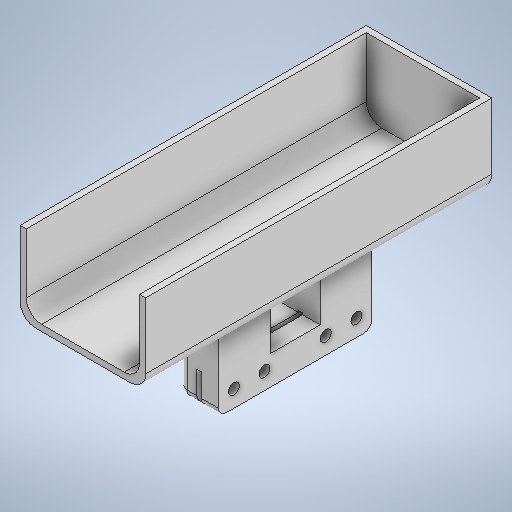
# Autodesk Inventor part: Battery and Rotation Sensor Holder
Saved by Autodesk Inventor 2025.1 (Build 291241020, 241B)
## iProperties
Created: 2024-12-11
Part Number: Battery and Rotation Sensor Holder
Material: Generic
Document SubType Name: Modeling
Designer: AtuStem
Density: 1 g/cm^3
Appearance: Default
Author: AtuStem
Autodesk Inventor part; units mm, degrees
ref_plane "YZ Plane" through (0, 0, 0) normal (1, 0, 0) x (0, 1, 0)
ref_plane "XZ Plane" through (0, 0, 0) normal (0, 1, 0) x (-1, 0, 0)
ref_plane "XY Plane" through (0, 0, 0) normal (0, 0, 1) x (1, 0, 0)
sketch "Sketch1" plane through (0, 0, 0) normal (1, 0, 0) x (0, 1, 0)
  line L0 (0, 0) -> (0, -12.7)
  circle A0 centre (0, -12.7) radius 3.9624
  line L1 (-6.985, -31.75) -> (5.08, -31.75)
  line L2 (5.08, -31.75) -> (5.08, 0)
  line L3 (5.08, 0) -> (-6.985, 0)
  line L4 (-6.985, 0) -> (-6.985, -31.75)
  circle A1 centre (0, -25.4) radius 3.9624
  line L5 (5.08, -10.3505) -> (29.6164, -10.3505)
  line L6 (29.6164, -10.3505) -> (29.6164, -31.75)
  line L7 (29.6164, -31.75) -> (5.08, -31.75)
  line L8 (5.08, -31.75) -> (5.08, -10.3505)
  line L9 (29.6164, -71.755) -> (27.0764, -71.755)
  line L10 (27.0764, -71.755) -> (27.0764, 0)
  line L11 (27.0764, 0) -> (29.6164, 0)
  line L12 (29.6164, 0) -> (29.6164, -71.755)
  line L13 (0, 0) -> (0, 12.7)
  circle A2 centre (0, 12.7) radius 3.9624
  line L14 (-6.985, 31.75) -> (5.08, 31.75)
  line L15 (5.08, 31.75) -> (5.08, 0)
  line L16 (-6.985, 0) -> (-6.985, 31.75)
  circle A3 centre (0, 25.4) radius 3.9624
  line L17 (5.08, 10.3505) -> (29.6164, 10.3505)
  line L18 (29.6164, 10.3505) -> (29.6164, 31.75)
  line L19 (29.6164, 31.75) -> (5.08, 31.75)
  line L20 (5.08, 31.75) -> (5.08, 10.3505)
  line L21 (29.6164, 71.755) -> (27.0764, 71.755)
  line L22 (27.0764, 71.755) -> (27.0764, 0)
  line L23 (29.6164, 0) -> (29.6164, 71.755)
  circle A4 centre (0, -25.4) radius 2.286
  circle A5 centre (0, -12.7) radius 2.286
  circle A6 centre (0, 12.7) radius 2.286
  circle A7 centre (0, 25.4) radius 2.286
  point P0 (27.0764, -31.75)
  point P1 (27.0764, -10.3505)
  point P2 (27.0764, 10.3505)
  point P3 (27.0764, 31.75)
  point P4 (28.3464, 0)
  point P5 (28.3464, -71.755)
  dimension "d0" = 12.7
  dimension "d1" = 7.9248
  dimension "d3" = 6.985
  dimension "d4" = 5.08
  dimension "d5" = 7.9248
  dimension "d6" = 12.7
  dimension "d7" = 6.35
  dimension "d8" = 10.3505
  dimension "d9" = 24.5364
  dimension "d11" = 2.54
  dimension "d31" = 4.572
  dimension "d32" = 4.572
  dimension "d33" = 4.572
  dimension "d34" = 4.572
  dimension "d46" = 71.755
  dimension "d47" = 0
  constraints: 48 end point, 11 symmetric about line, 8 centre point, 6 coincident, 6 parallel, 3 horizontal, 3 perpendicular, 2 midpoint, 2 point on line, 1 vertical, 2 other
  measures "d0" distance of L0.start L0.end
  measures "d1" diameter of A0
  measures "d3" distance from line of L4 L0.end
  measures "d4" distance from line of L2 L0.end
  measures "d5" diameter of A1
  measures "d6" distance of A1.centre L0.end
  measures "d7" distance from line of L1 A1.centre
  measures "d8" distance between parallel lines of L3 L5
  measures "d9" distance of L5.start L5.end
  measures "d11" distance of L9.start L9.end
  measures "d31" diameter of A4
  measures "d32" diameter of A6
  measures "d33" diameter of A7
  measures "d34" diameter of A5
  measures "d46" distance of point (28.346, 0) point (28.346, -71.755)
  measures "d47" distance between parallel lines of L3 L11
extrude "Extrusion1" add sketch "Sketch1" along normal blind 16.2306 contours A0 | L4 L3 L2 L1 | L2 L5 L10 L7 | L16 L14 L15 L3 | L19 L22 L17 L15 | A1 | A2 | A3 | A4 | A5 | A6 | A7
extrude "Extrusion2" add sketch "Sketch1" along normal mid plane 52.0446 contours L10 L5 L6 L7 | L7 L12 L9 L10 | L10 L11 L12 L5 | L22 L17 L23 L11 | L22 L21 L23 L19 | L19 L18 L17 L22
extrude "Extrusion3" cut sketch "Sketch1" along normal blind 2.54 contours A0 | A1 | A2 | A3 | A4 | A5 | A6 | A7
extrude "Extrusion4" cut sketch "Sketch1" along normal up to surface (16.2306 mm away) contours A4 | A5 | A6 | A7
sketch "Sketch3" plane through (0, -6.985, 31.75) normal (0, 0, 1) x (1, 0, 0)
  line L0 (0, 0) -> (16.2306, 0) projected
  line L1 (7.2644, 0) -> (8.9662, 0)
  line L2 (8.9662, 0) -> (8.9662, 12.7)
  line L3 (8.9662, 12.7) -> (7.2644, 12.7)
  line L4 (7.2644, 12.7) -> (7.2644, 0)
  line L5 (16.2306, 34.0614) -> (16.2306, 0) projected
  line L6 (0, 34.0614) -> (0, 0) projected
  point P0 (0, 6.985)
  dimension "d37" = 1.7018
  dimension "d38" = 12.7
  dimension "d39" = 16.2306
  dimension "d40" = 7.2644
  dimension "d41" = 7.2644
  constraints: 8 end point, 2 parallel, 1 horizontal, 1 perpendicular, 1 point on line
  measures "d37" distance between parallel lines of L2 L4
  measures "d38" distance of L1.end L2.end
  measures "d39" distance between parallel lines of L5 L6
  measures "d40" distance between parallel lines of L5 L2
  measures "d41" distance between parallel lines of L4 L6
extrude "Extrusion5" cut sketch "Sketch3" against normal up to surface (63.5 mm away)
fillet "Fillet1" radius 3.175 7 edges at (3.6322, -6.985, -31.75) (12.5984, -6.985, -31.75) (3.6322, -6.985, 31.75) (12.5984, -6.985, 31.75) (0, -6.985, 0) (0, 10.0457, -31.75) (0, 10.0457, 31.75)
sketch "Sketch4" plane through (-26.0223, 29.6164, 71.755) normal (0, 1, 0) x (1, 0, 0)
  line L0 (0, 143.51) -> (0, 0) projected
  line L1 (52.0446, 143.51) -> (0, 143.51)
  line L2 (0, 143.51) -> (0, 140.97)
  line L3 (0, 140.97) -> (52.0446, 140.97)
  line L4 (52.0446, 140.97) -> (52.0446, 143.51)
  line L5 (0, 0) -> (52.0446, 0) projected
  line L6 (0, 143.51) -> (2.54, 143.51)
  line L7 (2.54, 143.51) -> (2.54, 0)
  line L8 (2.54, 0) -> (0, 0)
  line L9 (0, 0) -> (0, 143.51)
  line L10 (52.0446, 143.51) -> (49.5046, 143.51)
  line L11 (49.5046, 143.51) -> (49.5046, 0)
  line L12 (49.5046, 0) -> (52.0446, 0)
  line L13 (52.0446, 0) -> (52.0446, 143.51)
  point P0 (26.0223, 71.755)
  point P1 (49.5046, 140.97)
  point P2 (2.54, 140.97)
  dimension "d48" = 2.54
  dimension "d51" = 2.54
  dimension "d52" = 2.54
  constraints: 24 end point, 6 parallel, 3 horizontal, 3 perpendicular, 3 point on line
  measures "d48" distance between parallel lines of L3 L1
  measures "d51" distance between parallel lines of L7 L0
  measures "d52" distance between parallel lines of L13 L11
extrude "Extrusion6" add sketch "Sketch4" along normal blind 31.115 contours L1 L7 L3 L0 | L3 L7 L5 L0 | L1 L11 L3 L7 | L1 L4 L3 L11 | L3 L13 L5 L11
fillet "Fillet2" radius 6.35 1 edges at (-23.4823, 29.6164, 1.27)
fillet "Fillet3" radius 6.35 1 edges at (23.4823, 29.6164, 1.27)
fillet "Fillet4" radius 6.35 2 edges at (-26.0223, 27.0764, 0) (26.0223, 27.0764, 0)
body "Solid1"
